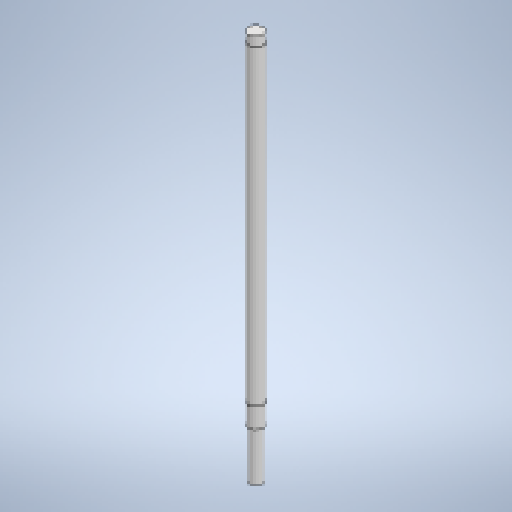
# Autodesk Inventor part: TRM 028 main shaft
Saved by Autodesk Inventor 2025 (Build 290162010, 162A)
## iProperties
Created: 2024-09-08
Part Number: TRM 028 main shaft
Material: Generic
Document SubType Name: Modeling
Designer: admin
Density: 1 g/cm^3
Appearance: Default
Mass: 304.342 g
Surface Area: 496.764 cm^2
Volume: 304.342 cm^3
Author: admin
Autodesk Inventor part; units mm, degrees
ref_plane "YZ Plane" through (0, 0, 0) normal (1, 0, 0) x (0, 1, 0)
ref_plane "XY Plane" through (0, 0, 0) normal (0, 0, 1) x (1, 0, 0)
sketch "Sketch1" plane through (0, 0, 0) normal (0, 1, 0) x (-1, 0, 0)
  line L0 (0, 0) -> (0, 280)
  line L1 (0, 280) -> (-12.5, 280)
  line L2 (-12.5, 280) -> (-12.5, 0)
  line L3 (-12.5, 0) -> (-12.5, -395)
  line L4 (-12.5, -395) -> (0, -395)
  line L5 (0, -395) -> (0, 0)
  line L6 (-9, -395) -> (-9, -310)
  line L7 (-9, -310) -> (-12.5, -310)
  line L8 (-12.5, -275) -> (-12, -275)
  line L9 (-12, -275) -> (-12, -310)
  line L10 (-12, 280) -> (-12, 265)
  line L11 (-12, 265) -> (-12.5, 265)
  dimension "d0" = 25
  dimension "d1" = 280
  dimension "d2" = 395
  dimension "d4" = 85
  dimension "d5" = 18
  dimension "d6" = 24
  dimension "d7" = 35
  dimension "d8" = 15
  constraints: 24 end point, 9 perpendicular, 8 point on line, 1 collinear, 1 horizontal alignment, 1 parallel, 1 vertical
  measures "d0" diameter of L2 L0
  measures "d1" distance of L1.end L2.end
  measures "d2" distance of L2.end L3.end
  measures "d4" distance of L6.start L6.end
  measures "d5" diameter of L6 L5
  measures "d6" diameter of L9 L5
  measures "d7" distance of L8.end L9.end
  measures "d8" distance of L10.start L10.end
revolve "Revolution1" add sketch "Sketch1" angle 360 about axis through (0, 0, 0) along (0, 0, 1) contours L5 L4 L6 L7 L9 L8 L3 L2 L11 L10 L1 L0
ref_plane "Work Plane1" through (0, 9, -352.5) normal (0, 1, 0) x (-1, 0, 0)
sketch "Sketch2" plane through (0, 9, -352.5) normal (0, 1, 0) x (-1, 0, 0)
  line L0 (9, -42.5) -> (-9, -42.5) projected
  line L1 (9, 42.5) -> (-9, 42.5) projected
  line L2 (9, -42.5) -> (9, 42.5) projected
  line L3 (-9, -42.5) -> (-9, 42.5) projected
  line L4 (9, -40.905) -> (-9, -40.905) construction
  line L5 (9, 37.095) -> (-9, 37.095) construction
  line L6 (0, 29.595) -> (0, -33.405) construction
  line L7 (-3, 26.595) -> (-3, -30.405)
  line L8 (3, -30.405) -> (3, 26.595)
  arc A0 (3, 26.595) -> (-3, 26.595) centre (0, 26.595) ccw
  arc A1 (-3, -30.405) -> (3, -30.405) centre (0, -30.405) ccw
  line L9 (0, 37.095) -> (0, -40.905) construction
  point P0 (0, 352.5)
  point P1 (0, -1.905)
  point P2 (0, -1.905)
  dimension "d9" = 1.595
  dimension "d10" = 78
  dimension "d11" = 63
  dimension "d12" = 6
  constraints: 14 end point, 6 point on circle, 6 point on line, 4 midpoint, 4 tangent, 2 centre point, 2 perpendicular, 1 coincident, 1 parallel, 1 vertical
  measures "d9" distance between parallel lines of L0 L4
  measures "d10" distance between parallel lines of L5 L4
  measures "d11" distance of L6.start L6.end
  measures "d12" diameter of A1
extrude "Extrusion1" cut sketch "Sketch2" against normal blind 3.5 contours A0 L8 A1 L7
chamfer "Chamfer1" distance 1 angle 45 3 edges at (-9, 0, -395) (-12, 0, 280) (-12, 0, -310)
body "Solid1"
